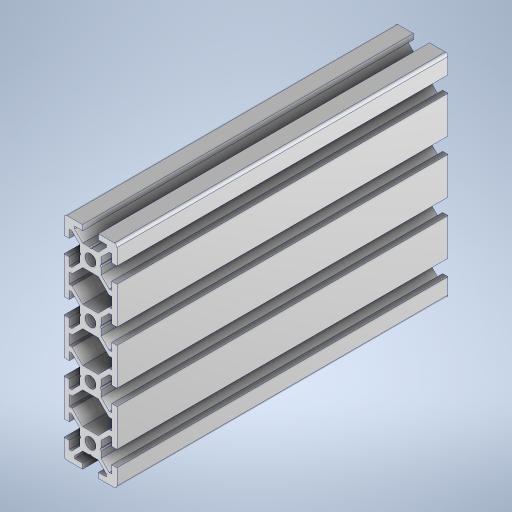
# Autodesk Inventor part: 2080 Z-column Support
Saved by Autodesk Inventor 2024 (Build 280153000, 153)
## iProperties
Category: PARTsolutions
Company: MISUMI
Created: 2024-12-14
Part Number: 2080 Z-column Support
Material: Aluminum 6061
Catalog Web Link: www.cadenas.de
Description: HFS5-2060, HFS5-2080, HFS5-4060, HFS5-4080, NFS5-2060, NFS5-2080, NFS5-4060, NFS5-4080-HFS5 Series Aluminum Extrusions 20mm Square -3 or more slots-
Vendor: MISUMI
Document SubType Name: Modeling
Designer: psAdmin
Manufacturer: MISUMI
Mass: 75.8441 g
Surface Area: 758.003 cm^2
Volume: 75.8441 cm^3
Density: 2.7 g/cm^3
Appearance: Aluminum - Flat
PSOL_IDENT_0: {$CADENAS_DATA/23d-libs/misumi/metric/38_al_extrusions_blackets/5/hfs5_2060.prj},622 {VTYP=3D},{NB=H
PSOL_IDENT_1: FS5-2080-125},{LINA=HFS5-2080-125},{NN=HFS5-2060, HFS5-2080, HFS5-4060, HFS5-4080, NFS5-2060, NFS5-2
PSOL_IDENT_2: 080, NFS5-4060, NFS5-4080},{DATE=08.05.2023 08:44:46},{GEOMDATE=27.07.2021 03:20:00},{VERSION=},{LIN
PSOL_IDENT_3: EID=200},{WBVAR=L,ALT1,ALT2,ALT4,ALT5,CP5,DL5,DR5,ALT6,ALT9,ALT10,ALT11,HP6,NHL6,DL6,NHR6,DR6,ALT7,A
PSOL_IDENT_4: LT8,NH9,AH,BH,CH,DH,EH,NH10,AV,BV,CV,DV,EV,NH11,AP,BP,CP,DP,EP,ALT12,ALT13,Z,NH12,XA,XB,XC,XD,XE,NH1
PSOL_IDENT_5: 3,YA,YB,YC,YD,YE,ALT16,HP16,DL16,DR16,ALT17,HQ17,JLP,ALT18,HQ18,KLP,ALT20},{WBNUMERIC=L,NH9,AH,BH,CH
PSOL_IDENT_6: ,DH,EH,NH10,AV,BV,CV,DV,EV,NH11,AP,BP,CP,DP,EP,NH12,XA,XB,XC,XD,XE,NH13,YA,YB,YC,YD,YE,HQ17,JLP,HQ18
PSOL_IDENT_7: ,KLP}  {NB=HFS5-2080-125},{LINA=HFS5-2080-125},{KT=DUMMY},{PN=HFS5-2080-125},{TPS=HFS5-2080},{MAT=A6
PSOL_IDENT_8: N01SS-T5 Aluminum Alloy},{ST=Clear Anodize},{FRMW=20},{FRMH=80},{FRD=4.2},{L=125},{MASS=1.64},{SA=60
PSOL_IDENT_9: 5},{LX=2.56x10^4},{LY=36.0x10^4},{ALT1=},{M1=0},{DPL1=0},{DPR1=0},{ALT1PN=},{ALT2=},{ALT2ALG= '','w/
PSOL_IDENT_10: o End Tapping (Heli-Coil Insert)','LHP','with LHP (Tapping on the Left (Heli-Coil Insert))','RHP','w
PSOL_IDENT_11: ith RHP (Tapping on the Right (Heli-Coil Insert))','HPW','with HPW (Tapping on Both Ends (Heli-Coil
PSOL_IDENT_12: Insert))' },{M2=0},{DP2=0},{ALT2PN=},{ALT4=},{ALT4ALG= '', 'w/o SC (High Precision Cut)', 'SC', 'wit
PSOL_IDENT_13: h SC (High Precision Cut)' },{ALT4PN=},{ALT5=},{ALT5ALG= '','w/o 45 Degree Cut','1','with 45 Degree
PSOL_IDENT_14: Cut' },{CP5=},{CP5ALG= '','N/A' },{DL5=},{DL5ALG= '','N/A' },{DR5=},{DR5ALG= '','N/A' },{FRMLALT5=0}
PSOL_IDENT_15: ,{FRMRALT5=0},{ALT5PN=},{ALT6=},{ALT6ALG= '','w/o Fastening Location Wrench Access Hole Alterations'
PSOL_IDENT_16: ,'1','with Fastening Location Wrench Access Hole Alterations' },{ALT9=},{ALT9ALG= '','w/o Location S
PSOL_IDENT_17: pecified Wrench Access Hole Alteratons (Horizontal)','1','with Location Specified Wrench Access Hole
PSOL_IDENT_18: Alteratons (Horizontal)' },{ALT10=},{ALT10ALG= '','w/o Location Specified Wrench Access Hole Altera
PSOL_IDENT_19: tons (Vertical)','1','with Location Specified Wrench Access Hole Alteratons (Vertical)' },{ALT11=},{
PSOL_IDENT_20: ALT11ALG= '','w/o Location Specified Wrench Access Hole Alteratons (Crisscross)','1','with Location
PSOL_IDENT_21: Specified Wrench Access Hole Alteratons (Crisscross)' },{DD6=0.00},{DD6ALG=0},{HP6=},{HP6ALG= '','N/
PSOL_IDENT_22: A' },{NHL6=},{NHL6ALG= '','N/A' },{DL6=},{DL6ALG= '','N/A' },{NHR6=},{NHR6ALG= '','N/A' },{DR6=},{DR
PSOL_IDENT_23: 6ALG= '','N/A' },{DD6PN=},{HL6=0},{HL6D=0},{HR6=0},{HR6D=0},{J6=0},{J6D=0},{K6=0},{K6D=0},{ALT7=},{A
PSOL_IDENT_24: LT7ALG= '','N/A' },{ALT8=},{ALT8ALG= '','N/A' },{ALT678PN=},{NH9=0},{NH9MAX=5},{NH9ALG=[0]},{AH=0.0}
PSOL_IDENT_25: ,{AHMIN=7},{AHMAX=120},{AHALG=[0]},{BH=0.0},{BHMIN=2},{BHMAX=122},{BHALG=[0]},{CH=0.0},{CHMIN=2},{CH
PSOL_IDENT_26: MAX=124},{CHALG=[0]},{DH=0.0},{DHMIN=2},{DHMAX=126},{DHALG=[0]},{EH=0.0},{EHMIN=2},{EHMAX=118},{EHAL
PSOL_IDENT_27: G=[0]},{NH10=0},{NH10MAX=5},{NH10ALG=[0]},{AV=0.0},{AVMIN=7},{AVMAX=120},{AVALG=[0]},{BV=0.0},{BVMIN=
PSOL_IDENT_28: 2},{BVMAX=122},{BVALG=[0]},{CV=0.0},{CVMIN=2},{CVMAX=124},{CVALG=[0]},{DV=0.0},{DVMIN=2},{DVMAX=126}
PSOL_IDENT_29: ,{DVALG=[0]},{EV=0.0},{EVMIN=2},{EVMAX=118},{EVALG=[0]},{NH11=0},{NH11MAX=5},{NH11ALG=[0]},{AP=0.0},
PSOL_IDENT_30: {APMIN=7},{APMAX=120},{APALG=[0]},{BP=0.0},{BPMIN=2},{BPMAX=122},{BPALG=[0]},{CP=0.0},{CPMIN=2},{CPM
PSOL_IDENT_31: AX=124},{CPALG=[0]},{DP=0.0},{DPMIN=2},{DPMAX=126},{DPALG=[0]},{EP=0.0},{EPMIN=2},{EPMAX=118},{EPALG=
PSOL_IDENT_32: [0]},{ALT9PN=},{ALT10PN=},{ALT11PN=},{ALT91011PN=},{ALT12=},{ALT12ALG= '','w/o Counterbore Hole in S
PSOL_IDENT_33: pecified Position (Vertical)','1','with Counterbore Hole in Specified Position (Vertical)' },{ALT13=
PSOL_IDENT_34: },{ALT13ALG= '','w/o Counterbore Hole in Specified Position (Horizontal)','1','with Counterbore Hole
PSOL_IDENT_35: in Specified Position (Horizontal)' },{Z=},{ZALG= '','N/A' },{DD12=0.0},{DD112=0.0},{NH12=0},{NH12M
PSOL_IDENT_36: AX=5},{NH12ALG=[0]},{XA=0.0},{XAMIN=7},{XAMAX=120},{XAALG=[0]},{XB=0.0},{XBMIN=2},{XBMAX=122},{XBALG=
PSOL_IDENT_37: [0]},{XC=0.0},{XCMIN=2},{XCMAX=124},{XCALG=[0]},{XD=0.0},{XDMIN=2},{XDMAX=126},{XDALG=[0]},{XE=0.0},
PSOL_IDENT_38: {XEMIN=2},{XEMAX=118},{XEALG=[0]},{NH13=0},{NH13MAX=5},{NH13ALG=[0]},{YA=0.0},{YAMIN=7},{YAMAX=120},
PSOL_IDENT_39: {YAALG=[0]},{YB=0.0},{YBMIN=2},{YBMAX=122},{YBALG=[0]},{YC=0.0},{YCMIN=2},{YCMAX=124},{YCALG=[0]},{Y
PSOL_IDENT_40: D=0.0},{YDMIN=2},{YDMAX=126},{YDALG=[0]},{YE=0.0},{YEMIN=2},{YEMAX=118},{YEALG=[0]},{ALT12PN=},{ALT1
PSOL_IDENT_41: 3PN=},{ALT1213PN=},{ALT16=},{ALT16ALG= '','w/o M Type Hole Alteration','1','with M Type Hole Alterat
PSOL_IDENT_42: ion' },{HP16=},{HP16ALG= '','N/A' },{DL16=},{DL16ALG= '','N/A' },{DR16=},{DR16ALG= '','N/A' },{H116=
PSOL_IDENT_43: 0},{D16=0.0},{ALT16PN=},{ALT17=},{ALT17ALG= '','w/o L Type Hole Alteration (Top)','1','with L Type H
PSOL_IDENT_44: ole Alteration (Top)' },{HQ17=0},{HQ17ALG=0},{JLP=0},{JLPMIN=4.9},{JLPMAX=0},{JLPALG=[0]},{L17=0},{D
PSOL_IDENT_45: 17=0.0},{ALT17PN=},{ALT18=},{ALT18ALG= '','w/o L Type Hole Alteration (Bottom)','1','with L Type Hol
PSOL_IDENT_46: e Alteration (Bottom)' },{HQ18=0},{HQ18ALG=0},{KLP=0},{KLPMIN=4.9},{KLPMAX=0},{KLPALG=[0]},{L18=0},{
PSOL_IDENT_47: D18=0.0},{ALT18PN=},{ALT20=},{ALT20PN=},{ERRORALT01=OK},{ERRORALT02=OK},{ERRORALT05=OK},{ERRORALT060
PSOL_IDENT_48: 91=OK},{ERRORALT06092=OK},{ERRORALT06093=OK},{ERRORALT06094=OK},{ERRORALT06101=OK},{ERRORALT06102=OK
PSOL_IDENT_49: },{ERRORALT06103=OK},{ERRORALT06104=OK},{ERRORALT06111=OK},{ERRORALT06112=OK},{ERRORALT06113=OK},{ER
PSOL_IDENT_50: RORALT06114=OK},{ERRORALT06121=OK},{ERRORALT06122=OK},{ERRORALT06123=OK},{ERRORALT06124=OK},{ERRORAL
PSOL_IDENT_51: T06131=OK},{ERRORALT06132=OK},{ERRORALT06133=OK},{ERRORALT06134=OK},{ERRORALT0616=OK},{ERRORALT06171=
PSOL_IDENT_52: OK},{ERRORALT06172=OK},{ERRORALT06173=OK},{ERRORALT06181=OK},{ERRORALT06182=OK},{ERRORALT06183=OK},{
PSOL_IDENT_53: ERRORALT0911=OK},{ERRORALT0913=OK},{ERRORALT0916=OK},{ERRORALT0917=OK},{ERRORALT0918=OK},{ERRORALT10
PSOL_IDENT_54: 11=OK},{ERRORALT1012=OK},{ERRORALT1016=OK},{ERRORALT1017=OK},{ERRORALT1018=OK},{ERRORALT1112=OK},{ER
PSOL_IDENT_55: RORALT1113=OK},{ERRORALT1116=OK},{ERRORALT1117=OK},{ERRORALT1118=OK},{ERRORALT1216=OK},{ERRORALT1217=
PSOL_IDENT_56: OK},{ERRORALT1218=OK},{ERRORALT1316=OK},{ERRORALT1317=OK},{ERRORALT1318=OK},{ERRORALT1617=OK},{ERROR
PSOL_IDENT_57: ALT1618=OK},{ERRORPN=},{TFW=0}
NB: HFS5-2080-125
NN: HFS5-2060, HFS5-2080, HFS5-4060, HFS5-4080, NFS5-2060, NFS5-2080, NFS5-4060, NFS5-4080
NT: HFS5 Series Aluminum Extrusions 20mm Square -3 or more slots-
NBSYN: $PN.
LINA: HFS5-2080-125
CATALOG: Misumi
PN: HFS5-2080-125
TPS: HFS5-2080
MAT: A6N01SS-T5 Aluminum Alloy
ST: Clear Anodize
L: 125
MASS: 1.64
SA: 605
LX: 2.56x10^4
LY: 36.0x10^4
ALT1: w/o End Tapping
M1: 0
DPL1: 0
DPR1: 0
ALT2: w/o End Tapping (Heli-Coil Insert)
M2: 0
DP2: 0
ALT4: w/o SC (High Precision Cut)
ALT5: w/o 45 Degree Cut
CP5: N/A
DL5: N/A
DR5: N/A
ALT6: w/o Fastening Location Wrench Access Hole Alterations
ALT9: w/o Location Specified Wrench Access Hole Alteratons (Horizontal)
ALT10: w/o Location Specified Wrench Access Hole Alteratons (Vertical)
ALT11: w/o Location Specified Wrench Access Hole Alteratons (Crisscross)
DD6: 0
HP6: N/A
NHL6: N/A
DL6: N/A
NHR6: N/A
DR6: N/A
HL6D: 0
HR6D: 0
J6D: 0
K6D: 0
ALT7: N/A
ALT8: N/A
NH9: 0
AH: 0
BH: 0
CH: 0
DH: 0
EH: 0
NH10: 0
AV: 0
BV: 0
CV: 0
DV: 0
EV: 0
NH11: 0
AP: 0
BP: 0
CP: 0
DP: 0
EP: 0
ALT12: w/o Counterbore Hole in Specified Position (Vertical)
ALT13: w/o Counterbore Hole in Specified Position (Horizontal)
Z: N/A
DD12: 0
DD112: 0
NH12: 0
XA: 0
XB: 0
XC: 0
XD: 0
XE: 0
NH13: 0
YA: 0
YB: 0
YC: 0
YD: 0
YE: 0
ALT16: w/o M Type Hole Alteration
HP16: N/A
DL16: N/A
DR16: N/A
H116: 0
D16: 0
ALT17: w/o L Type Hole Alteration (Top)
HQ17: 0
JLP: 0
D17: 0
ALT18: w/o L Type Hole Alteration (Bottom)
HQ18: 0
KLP: 0
D18: 0
ALT20: w/o CW (End Face C Chamfering)
SUPPLIER: MISUMI
ARTICLENO: HFS5-2080-125
BOMINFO: HFS5-2080-125
CREATOR: CADENAS GmbH
Title: HFS5-2080-125
Author: Cadenas PARTsolutions
Comments: HFS5 Series Aluminum Extrusions 20mm Square -3 or more slots-
Autodesk Inventor part; units mm, degrees
ref_plane "YZ Plane" through (0, 0, 0) normal (1, 0, 0) x (0, 1, 0)
ref_plane "XZ Plane" through (0, 0, 0) normal (0, 1, 0) x (-1, 0, 0)
ref_plane "XY Plane" through (0, 0, 0) normal (0, 0, 1) x (1, 0, 0)
sketch "Sketch_1" plane through (0, 0, 0) normal (0, 0, 1) x (1, 0, 0)
  arc A0 (-10, -39) -> (-9, -40) centre (-9, -39) ccw
  line L0 (-9, -40) -> (-3, -40)
  line L1 (-3, -40) -> (-3, -38)
  line L2 (-3, -38) -> (-6, -38)
  line L3 (-6, -38) -> (-6, -37.0607)
  line L4 (-6, -37.0607) -> (-2.9393, -34)
  line L5 (-2.9393, -34) -> (-0.5196, -34)
  line L6 (-0.5196, -34) -> (0, -33.7)
  line L7 (0, -33.7) -> (0.5196, -34)
  line L8 (0.5196, -34) -> (2.9393, -34)
  line L9 (2.9393, -34) -> (6, -37.0607)
  line L10 (6, -37.0607) -> (6, -38)
  line L11 (6, -38) -> (3, -38)
  line L12 (3, -38) -> (3, -40)
  line L13 (3, -40) -> (9, -40)
  arc A1 (9, -40) -> (10, -39) centre (9, -39) ccw
  line L14 (10, -39) -> (10, -33)
  line L15 (10, -33) -> (8, -33)
  line L16 (8, -33) -> (8, -36)
  line L17 (8, -36) -> (7.0607, -36)
  line L18 (7.0607, -36) -> (4, -32.9393)
  line L19 (4, -32.9393) -> (4, -30.5196)
  line L20 (4, -30.5196) -> (3.7, -30)
  line L21 (3.7, -30) -> (4, -29.4804)
  line L22 (4, -29.4804) -> (4, -27.0607)
  line L23 (4, -27.0607) -> (7.0607, -24)
  line L24 (7.0607, -24) -> (8, -24)
  line L25 (8, -24) -> (8, -27)
  line L26 (8, -27) -> (10, -27)
  line L27 (10, -27) -> (10, -13)
  line L28 (10, -13) -> (8, -13)
  line L29 (8, -13) -> (8, -16)
  line L30 (8, -16) -> (7.0607, -16)
  line L31 (7.0607, -16) -> (4, -12.9393)
  line L32 (4, -12.9393) -> (4, -10.5196)
  line L33 (4, -10.5196) -> (3.7, -10)
  line L34 (3.7, -10) -> (4, -9.4804)
  line L35 (4, -9.4804) -> (4, -7.0607)
  line L36 (4, -7.0607) -> (7.0607, -4)
  line L37 (7.0607, -4) -> (8, -4)
  line L38 (8, -4) -> (8, -7)
  line L39 (8, -7) -> (10, -7)
  line L40 (10, -7) -> (10, 7)
  line L41 (10, 7) -> (8, 7)
  line L42 (8, 7) -> (8, 4)
  line L43 (8, 4) -> (7.0607, 4)
  line L44 (7.0607, 4) -> (4, 7.0607)
  line L45 (4, 7.0607) -> (4, 9.4804)
  line L46 (4, 9.4804) -> (3.7, 10)
  line L47 (3.7, 10) -> (4, 10.5196)
  line L48 (4, 10.5196) -> (4, 12.9393)
  line L49 (4, 12.9393) -> (7.0607, 16)
  line L50 (7.0607, 16) -> (8, 16)
  line L51 (8, 16) -> (8, 13)
  line L52 (8, 13) -> (10, 13)
  line L53 (10, 13) -> (10, 27)
  line L54 (10, 27) -> (8, 27)
  line L55 (8, 27) -> (8, 24)
  line L56 (8, 24) -> (7.0607, 24)
  line L57 (7.0607, 24) -> (4, 27.0607)
  line L58 (4, 27.0607) -> (4, 29.4804)
  line L59 (4, 29.4804) -> (3.7, 30)
  line L60 (3.7, 30) -> (4, 30.5196)
  line L61 (4, 30.5196) -> (4, 32.9393)
  line L62 (4, 32.9393) -> (7.0607, 36)
  line L63 (7.0607, 36) -> (8, 36)
  line L64 (8, 36) -> (8, 33)
  line L65 (8, 33) -> (10, 33)
  line L66 (10, 33) -> (10, 39)
  arc A2 (10, 39) -> (9, 40) centre (9, 39) ccw
  line L67 (9, 40) -> (3, 40)
  line L68 (3, 40) -> (3, 38)
  line L69 (3, 38) -> (6, 38)
  line L70 (6, 38) -> (6, 37.0607)
  line L71 (6, 37.0607) -> (2.9393, 34)
  line L72 (2.9393, 34) -> (0.5196, 34)
  line L73 (0.5196, 34) -> (0, 33.7)
  line L74 (0, 33.7) -> (-0.5196, 34)
  line L75 (-0.5196, 34) -> (-2.9393, 34)
  line L76 (-2.9393, 34) -> (-6, 37.0607)
  line L77 (-6, 37.0607) -> (-6, 38)
  line L78 (-6, 38) -> (-3, 38)
  line L79 (-3, 38) -> (-3, 40)
  line L80 (-3, 40) -> (-9, 40)
  arc A3 (-9, 40) -> (-10, 39) centre (-9, 39) ccw
  line L81 (-10, 39) -> (-10, 33)
  line L82 (-10, 33) -> (-8, 33)
  line L83 (-8, 33) -> (-8, 36)
  line L84 (-8, 36) -> (-7.0607, 36)
  line L85 (-7.0607, 36) -> (-4, 32.9393)
  line L86 (-4, 32.9393) -> (-4, 30.5196)
  line L87 (-4, 30.5196) -> (-3.7, 30)
  line L88 (-3.7, 30) -> (-4, 29.4804)
  line L89 (-4, 29.4804) -> (-4, 27.0607)
  line L90 (-4, 27.0607) -> (-7.0607, 24)
  line L91 (-7.0607, 24) -> (-8, 24)
  line L92 (-8, 24) -> (-8, 27)
  line L93 (-8, 27) -> (-10, 27)
  line L94 (-10, 27) -> (-10, 13)
  line L95 (-10, 13) -> (-8, 13)
  line L96 (-8, 13) -> (-8, 16)
  line L97 (-8, 16) -> (-7.0607, 16)
  line L98 (-7.0607, 16) -> (-4, 12.9393)
  line L99 (-4, 12.9393) -> (-4, 10.5196)
  line L100 (-4, 10.5196) -> (-3.7, 10)
  line L101 (-3.7, 10) -> (-4, 9.4804)
  line L102 (-4, 9.4804) -> (-4, 7.0607)
  line L103 (-4, 7.0607) -> (-7.0607, 4)
  line L104 (-7.0607, 4) -> (-8, 4)
  line L105 (-8, 4) -> (-8, 7)
  line L106 (-8, 7) -> (-10, 7)
  line L107 (-10, 7) -> (-10, -7)
  line L108 (-10, -7) -> (-8, -7)
  line L109 (-8, -7) -> (-8, -4)
  line L110 (-8, -4) -> (-7.0607, -4)
  line L111 (-7.0607, -4) -> (-4, -7.0607)
  line L112 (-4, -7.0607) -> (-4, -9.4804)
  line L113 (-4, -9.4804) -> (-3.7, -10)
  line L114 (-3.7, -10) -> (-4, -10.5196)
  line L115 (-4, -10.5196) -> (-4, -12.9393)
  line L116 (-4, -12.9393) -> (-7.0607, -16)
  line L117 (-7.0607, -16) -> (-8, -16)
  line L118 (-8, -16) -> (-8, -13)
  line L119 (-8, -13) -> (-10, -13)
  line L120 (-10, -13) -> (-10, -27)
  line L121 (-10, -27) -> (-8, -27)
  line L122 (-8, -27) -> (-8, -24)
  line L123 (-8, -24) -> (-7.0607, -24)
  line L124 (-7.0607, -24) -> (-4, -27.0607)
  line L125 (-4, -27.0607) -> (-4, -29.4804)
  line L126 (-4, -29.4804) -> (-3.7, -30)
  line L127 (-3.7, -30) -> (-4, -30.5196)
  line L128 (-4, -30.5196) -> (-4, -32.9393)
  line L129 (-4, -32.9393) -> (-7.0607, -36)
  line L130 (-7.0607, -36) -> (-8, -36)
  line L131 (-8, -36) -> (-8, -33)
  line L132 (-8, -33) -> (-10, -33)
  line L133 (-10, -33) -> (-10, -39)
  line L134 (-8, 22) -> (-8, 18)
  line L135 (-8, 18) -> (-6.9393, 18)
  line L136 (-6.9393, 18) -> (-2.9393, 14)
  line L137 (-2.9393, 14) -> (2.9393, 14)
  line L138 (2.9393, 14) -> (6.9393, 18)
  line L139 (6.9393, 18) -> (8, 18)
  line L140 (8, 18) -> (8, 22)
  line L141 (8, 22) -> (6.9393, 22)
  line L142 (6.9393, 22) -> (2.9393, 26)
  line L143 (2.9393, 26) -> (-2.9393, 26)
  line L144 (-2.9393, 26) -> (-6.9393, 22)
  line L145 (-6.9393, 22) -> (-8, 22)
  line L146 (-8, -2) -> (-6.9393, -2)
  line L147 (-6.9393, -2) -> (-2.9393, -6)
  line L148 (-2.9393, -6) -> (2.9393, -6)
  line L149 (2.9393, -6) -> (6.9393, -2)
  line L150 (6.9393, -2) -> (8, -2)
  line L151 (8, -2) -> (8, 2)
  line L152 (8, 2) -> (6.9393, 2)
  line L153 (6.9393, 2) -> (2.9393, 6)
  line L154 (2.9393, 6) -> (-2.9393, 6)
  line L155 (-2.9393, 6) -> (-6.9393, 2)
  line L156 (-6.9393, 2) -> (-8, 2)
  line L157 (-8, 2) -> (-8, -2)
  line L158 (-8, -22) -> (-6.9393, -22)
  line L159 (-6.9393, -22) -> (-2.9393, -26)
  line L160 (-2.9393, -26) -> (2.9393, -26)
  line L161 (2.9393, -26) -> (6.9393, -22)
  line L162 (6.9393, -22) -> (8, -22)
  line L163 (8, -22) -> (8, -18)
  line L164 (8, -18) -> (6.9393, -18)
  line L165 (6.9393, -18) -> (2.9393, -14)
  line L166 (2.9393, -14) -> (-2.9393, -14)
  line L167 (-2.9393, -14) -> (-6.9393, -18)
  line L168 (-6.9393, -18) -> (-8, -18)
  line L169 (-8, -18) -> (-8, -22)
  constraints: 340 end point, 8 point on circle, 4 centre point
extrude "Extrusion1" add sketch "Sketch_1" along normal mid plane 125
sketch "Sketch2" plane through (0, 0, -62.5) normal (0, 0, -1) x (1, 0, 0)
  point P0 (0, 30)
hole "Hole1" at (0, -30, -62.5) direction (0, 0, 1) diameter 4.134 end through all thread size "M5x0.8" class "6H" standard "ANSI Metric M Profile"
pattern_linear "Rectangular Pattern1" count 4 spacing 20 along (0, 1, 0) of "Hole1"
mirror "Mirror1" about plane through (0, 0, 0) normal (0, 0, 1) of "Hole1", "Rectangular Pattern1"
body "Solid1"
